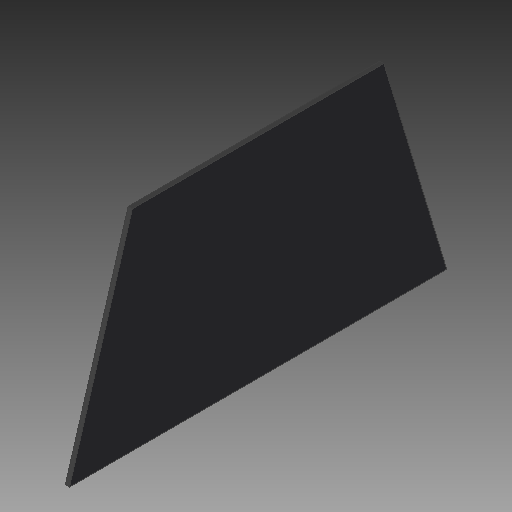
# Autodesk Inventor part: Trapezoid support plate
Saved by Autodesk Inventor 2019 (Build 230136000, 136)
## iProperties
Created: 2019-02-04
Part Number: Trapezoid support plate
Material: Generic
Document SubType Name: Modeling
Designer: josh
Density: 1 g/cm^3
Appearance: Default
Mass: 61.4515 g
Surface Area: 500.283 cm^2
Volume: 61.4515 cm^3
Author: josh
Autodesk Inventor part; units mm, degrees
ref_plane "YZ Plane" through (0, 0, 0) normal (1, 0, 0) x (0, 1, 0)
ref_plane "XZ Plane" through (0, 0, 0) normal (0, 1, 0) x (-1, 0, 0)
ref_plane "XY Plane" through (0, 0, 0) normal (0, 0, 1) x (1, 0, 0)
sketch "Sketch1" plane through (0, 0, 0) normal (1, 0, 0) x (0, 1, 0)
  line L0 (0, 0) -> (0, -228.6)
  line L1 (127, -114.3) -> (127, -190.5)
  line L2 (127, -114.3) -> (127, -38.1)
  line L3 (127, -38.1) -> (0, 0)
  line L4 (127, -190.5) -> (0, -228.6)
  dimension "d0" = 228.6
  dimension "d3" = 127
  constraints: 10 end point, 3 vertical
  measures "d0" distance of L0.start L0.end
  measures "d3" distance between parallel lines of L0 L2
extrude "Extrusion1" add sketch "Sketch1" along normal blind 2.54
body "Solid1"
